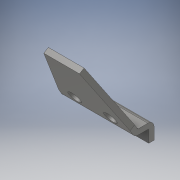
# Autodesk Inventor part: P-POD_DoorStop
Saved by Autodesk Inventor 2018 (Build 220112000, 112)
## iProperties
Created: 2018-07-16
Part Number: P-POD_DoorStop
Material: Aluminum 6061
Document SubType Name: Modeling
Designer: Bradley
Density: 2.7 g/cm^3
Appearance: Anodized - Light Gray
Author: Bradley
Autodesk Inventor part; units mm, degrees
ref_plane "YZ Plane" through (0, 0, 0) normal (1, 0, 0) x (0, 1, 0)
ref_plane "XZ Plane" through (0, 0, 0) normal (0, 1, 0) x (-1, 0, 0)
ref_plane "XY Plane" through (0, 0, 0) normal (0, 0, 1) x (1, 0, 0)
sketch "Sketch1" plane through (0, 0, 0) normal (1, 0, 0) x (0, 1, 0)
  line L0 (1.5, -5) -> (1.5, 5)
  line L1 (1.5, 5) -> (-7.7318, 5)
  line L2 (-9.4639, 2) -> (-1.5, 2)
  line L3 (-1.5, 2) -> (-1.5, -5)
  line L4 (-1.5, -5) -> (1.5, -5)
  line L5 (-7.7318, 5) -> (-27.7318, 39.641)
  line L6 (-27.7318, 39.641) -> (-30.3299, 38.141)
  line L7 (-30.3299, 38.141) -> (-9.4639, 2)
  point P0 (0, 0)
  point P1 (0, -5)
  point P2 (1.5, 0)
  dimension "d0" = 3
  dimension "d1" = 10
  dimension "d2" = 150
  dimension "d3" = 3
  dimension "d4" = 3
  dimension "d5" = 40
  dimension "d6" = 7.995
  constraints: 16 end point, 2 horizontal, 2 midpoint, 2 parallel, 2 perpendicular, 1 horizontal alignment, 1 vertical, 1 vertical alignment
  measures "d0" distance of L3.end L0.start
  measures "d1" distance of L0.start L0.end
  measures "d2" angle of L3 L5
  measures "d3" distance between parallel lines of L2 L1
  measures "d4" distance between parallel lines of L7 L5
  measures "d5" distance of L1.end L5.end
  measures "d6" distance from line of L5 L0.end
extrude "Extrusion1" add sketch "Sketch1" along normal mid plane 40
fillet "Fillet1" radius 3.5 2 edges at (0, 1.5, 5) (0, -9.4639, 2)
fillet "Fillet1" radius 0.5 2 edges at (0, -1.5, 2) (0, -7.7318, 5)
sketch "Sketch2" plane through (-20, -1.5, -5) normal (0, -1, 0) x (1, 0, 0)
  line L0 (30, 3.5) -> (10, 3.5) construction
  line L1 (0, 0) -> (40, 0) construction
  point P0 (20, 5)
  point P1 (20, 3.5)
  dimension "d11" = 20
  dimension "d12" = 3.5
  constraints: 2 coincident, 2 end point, 1 horizontal, 1 midpoint, 1 vertical alignment
  measures "d11" distance of L0.start L0.end
  measures "d12" distance between parallel lines of L0 L1
hole "Hole1" at (10, -1.5, -1.5) at (-10, -1.5, -1.5) direction (0, 1, 0) diameter 3.3 end through all
sketch "Sketch3" plane through (-20, -27.7318, 39.641) normal (0, 0.8660254, 0.5) x (1, 0, 0)
  line L0 (0, 39.7113) -> (40, 39.7113) projected
  line L1 (0, 0) -> (0, 39.7113) projected
  line L2 (0, 0) -> (40, 0) projected
  line L3 (40, 39.7113) -> (40, 0) projected
  line L4 (0, 0) -> (40, 0) projected
  line L5 (10, 0) -> (0, 36.7113)
  line L6 (0, 39.7113) -> (0, 0) projected
  line L7 (40, 36.7113) -> (30, 0)
  circle A0 centre (10, 34.7113) radius 3.5
  circle A1 centre (30, 34.7113) radius 3.5
  line L8 (10, 34.7113) -> (30, 34.7113) construction
  point P0 (20, 48.196)
  point P1 (20, 34.7113)
  point P2 (20, 0)
  dimension "d20" = 7
  dimension "d21" = 20
  dimension "d22" = 3
  dimension "d23" = 20
  dimension "d24" = 5
  constraints: 6 end point, 4 point on line, 2 centre point, 2 horizontal alignment, 2 midpoint, 1 equal length, 1 equal radius, 1 horizontal, 1 vertical alignment
  measures "d20" diameter of A0
  measures "d21" distance of L7.end L5.start
  measures "d22" distance from line of L5.end L0
  measures "d23" distance of L8.start L8.end
  measures "d24" distance between parallel lines of L8 L0
extrude "Extrusion2" cut sketch "Sketch3" against normal through all contours L5 L2 L1 | L3 L2 L7 | A0 | A1
equation "\"d3\" = d0"
equation "\"d4\" = d0"
body "Solid1"
